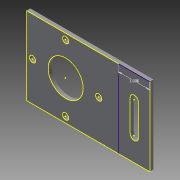
# Autodesk Inventor part: p80 mount plate
Saved by Autodesk Inventor 2013 (Build 170138000, 138)
## iProperties
Created: 2013-01-31
Part Number: p80 mount plate
Material: Generic
Document SubType Name: Sheet Metal
Designer: Arpan
Density: 1 g/cm^3
Sheet Metal Rule: Default
Author: Arpan
Autodesk Inventor part; units mm, degrees
ref_plane "YZ Plane" through (0, 0, 0) normal (1, 0, 0) x (0, 1, 0)
ref_plane "XZ Plane" through (0, 0, 0) normal (0, 1, 0) x (-1, 0, 0)
ref_plane "XY Plane" through (0, 0, 0) normal (0, 0, 1) x (1, 0, 0)
sketch "Sketch1" plane through (0, 0, 0) normal (0, 0, 1) x (1, 0, 0)
  line L0 (0, 0) -> (-63.5, 0)
  line L1 (-63.5, 0) -> (-63.5, 63.5)
  line L2 (-63.5, 63.5) -> (0, 63.5)
  circle A0 centre (-58.7502, 31.75) radius 2.54
  circle A1 centre (-31.75, 58.7502) radius 2.54
  circle A2 centre (-4.7498, 31.75) radius 2.54
  circle A3 centre (-31.75, 4.7498) radius 2.54
  line L3 (0, 63.5) -> (36.9316, 63.5)
  line L4 (36.9316, 63.5) -> (36.9316, 0)
  line L5 (36.9316, 0) -> (0, 0)
  circle A4 centre (-31.75, 31.75) radius 14.2875
  line L6 (36.9316, 63.5) -> (24.2316, 63.5)
  line L7 (24.2316, 63.5) -> (24.2316, 44.45)
  line L8 (24.2316, 44.45) -> (24.2316, 19.05)
  circle A5 centre (24.2316, 44.45) radius 3.3782
  circle A6 centre (24.2316, 19.05) radius 3.3782
  line L9 (20.8534, 44.45) -> (20.8534, 19.05)
  line L10 (27.6098, 19.05) -> (27.6098, 44.45)
  dimension "d0" = 63.5
  dimension "d1" = 63.5
  dimension "d6" = 5.08
  dimension "d7" = 5.08
  dimension "d8" = 5.08
  dimension "d9" = 5.08
  dimension "d11" = 36.9316
  dimension "d12" = 28.575
  dimension "d13" = 12.7
  dimension "d14" = 19.05
  dimension "d15" = 25.4
  dimension "d16" = 6.7564
  dimension "d17" = 6.7564
  measures "d0" distance of L0.start L0.end
  measures "d1" distance of L0.end L1.end
  measures "d6" diameter of A0
  measures "d7" diameter of A1
  measures "d8" diameter of A2
  measures "d9" diameter of A3
  measures "d11" distance of L2.end L3.end
  measures "d12" diameter of A4
  measures "d13" distance of L3.end L6.end
  measures "d14" distance of L6.end L7.end
  measures "d15" distance of L7.end L8.end
  measures "d16" diameter of A5
  measures "d17" diameter of A6
extrude "Plate2" add sketch "Sketch1" along normal blind 3.048 contours L0 L1 L2 L3 L4 L5 | L10 A6 L8 A5 | A5 L8 A6 L9
sketch "Sketch4" plane through (0, 0, 3.048) normal (0, 0, 1) x (1, 0, 0)
  circle A0 centre (24.2316, 19.05) radius 3.3782 projected
  circle A1 centre (24.2316, 44.45) radius 3.3782 projected
  line L0 (20.8534, 44.45) -> (20.8534, 19.05)
  line L1 (27.6098, 19.05) -> (27.6098, 44.45)
  point P0 (0, 0)
  constraints: 4 end point, 4 point on circle, 3 tangent
extrude "Cut1" cut sketch "Sketch4" against normal blind 3.048 contours A0 L0 A1 L1
sketch "Sketch5" plane through (0, 0, 3.048) normal (0, 0, 1) x (1, 0, 0)
  line L0 (36.9316, 0) -> (-63.5, 0) projected
  line L1 (36.9316, 63.5) -> (36.9316, 0) projected
  line L2 (-63.5, 63.5) -> (36.9316, 63.5) projected
  line L3 (-63.5, 0) -> (-63.5, 63.5) projected
  circle A0 centre (-58.7502, 31.75) radius 2.54 projected
  circle A1 centre (-31.75, 58.7502) radius 2.54 projected
  circle A2 centre (-4.7498, 31.75) radius 2.54 projected
  circle A3 centre (-31.75, 4.7498) radius 2.54 projected
  line L4 (20.8534, 19.05) -> (20.8534, 44.45) projected
  arc A4 (27.6098, 44.45) -> (20.8534, 44.45) centre (24.2316, 44.45) ccw projected
  line L5 (27.6098, 44.45) -> (27.6098, 19.05) projected
  arc A5 (20.8534, 19.05) -> (27.6098, 19.05) centre (24.2316, 19.05) ccw projected
  circle A6 centre (-31.75, 31.75) radius 14.2875 projected
  line L6 (36.9316, 63.5) -> (11.5316, 63.5)
  line L7 (11.5316, 63.5) -> (11.5316, 0)
  point P0 (0, 0)
  dimension "d21" = 25.4
  constraints: 4 end point, 2 point on line, 1 perpendicular
  measures "d21" distance of L1.start L6.end
equation "\"d19\" = Thickness"
equation "\"BendRadius\" = Thickness"
equation "\"BendReliefWidth\" = Thickness"
equation "\"BendReliefDepth\" = 0.5 * Thickness"
equation "\"CornerReliefSize\" = 4 * Thickness"
equation "\"MinimumRemnant\" = 2 * Thickness"
equation "\"TransitionRadius\" = BendRadius"
equation "\"JacobiRadiusSize\" = BendRadius"
equation "\"GapSize\" = Thickness"
equation "\"d10\" = BendRadius"
equation "\"d18\" = BendRadius"
equation "\"Thickness\" = 3.048"
body "Solid2"
